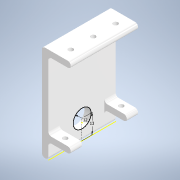
# Autodesk Inventor part: BearingBracket
Saved by Autodesk Inventor 2021 (Build 250183000, 183)
## iProperties
Created: 2021-05-21
Part Number: BearingBracket
Material: PC/ABS Plastic
Document SubType Name: Modeling
Designer: sami8
Density: 0.357273 g/cm^3
Appearance: Smooth - White
Author: sami8
Autodesk Inventor part; units mm, degrees
ref_plane "YZ Plane" through (0, 0, 0) normal (1, 0, 0) x (0, 1, 0)
ref_plane "XZ Plane" through (0, 0, 0) normal (0, 1, 0) x (-1, 0, 0)
ref_plane "XY Plane" through (0, 0, 0) normal (0, 0, 1) x (1, 0, 0)
sketch "Sketch1" plane through (0, 0, 0) normal (0, 0, 1) x (1, 0, 0)
  line L0 (0, 0) -> (15, 0)
  line L1 (15, 0) -> (15, 4)
  line L2 (15, 4) -> (0, 4)
  line L3 (0, 4) -> (0, 0)
  line L4 (0, 53.5) -> (15, 53.5)
  line L5 (15, 53.5) -> (15, 49.5)
  line L6 (15, 49.5) -> (0, 49.5)
  line L7 (0, 49.5) -> (0, 53.5)
  line L8 (0, 53.5) -> (-4.3, 53.5)
  line L9 (-4.3, 53.5) -> (-4.3, -10.5)
  line L10 (-4.3, -10.5) -> (0, -10.5)
  line L11 (0, -10.5) -> (0, 53.5)
  point P0 (0, 49.5)
  dimension "d0" = 15
  dimension "d1" = 4
  dimension "d2" = 15
  dimension "d3" = 4
  dimension "d4" = 45.5
  dimension "d5" = 4.3
  dimension "d6" = 64
  constraints: 24 end point, 6 parallel, 3 horizontal, 3 perpendicular, 1 point on line
  measures "d0" distance of L2.end L1.end
  measures "d1" distance of L1.end L0.end
  measures "d2" distance of L5.end L6.end
  measures "d3" distance of L4.end L5.end
  measures "d4" distance between parallel lines of L6 L2
  measures "d5" distance of L10.end L9.end
  measures "d6" distance between parallel lines of L8 L10
extrude "Extrusion1" add sketch "Sketch1" along normal mid plane 45
extrude "Extrusion2" cut sketch "Sketch1" along normal mid plane 30 contours L3 L2 L1 L0
sketch "Sketch3" plane through (0, 49.5, 22.5) normal (0, -1, 0) x (1, 0, 0)
  line L0 (0, 0) -> (15, 0) projected
  line L1 (7.5, 0) -> (7.5, -45)
  line L2 (15, -45) -> (0, -45) projected
  circle A0 centre (7.5, -3.75) radius 1.55
  circle A1 centre (7.5, -7.5) radius 1.55
  circle A2 centre (7.5, -22.5) radius 1.55
  circle A3 centre (7.5, -37.5) radius 1.55
  circle A4 centre (7.5, -41.25) radius 1.55
  line L3 (0, 0) -> (15, 0) projected
  line L4 (15, -45) -> (0, -45) projected
  line L5 (15, -45) -> (15, 0) projected
  point P0 (0, -22.5)
  dimension "d11" = 3.1
  dimension "d12" = 3.1
  dimension "d13" = 3.1
  dimension "d14" = 3.1
  dimension "d15" = 3.1
  dimension "d16" = 3.75
  dimension "d17" = 7.5
  dimension "d18" = 3.75
  dimension "d19" = 7.5
  dimension "d20" = 7.5
  constraints: 5 centre point, 4 point on line, 3 midpoint, 2 end point
  measures "d11" diameter of A0
  measures "d12" diameter of A1
  measures "d13" diameter of A2
  measures "d14" diameter of A3
  measures "d15" diameter of A4
  measures "d16" distance from line of L0 A0.centre
  measures "d17" distance from line of A1.centre L0
  measures "d18" distance from line of L2 A4.centre
  measures "d19" distance from line of L2 A3.centre
  measures "d20" distance between parallel lines of L5 L1
extrude "Extrusion3" cut sketch "Sketch3" along normal through all contours A0 L1 | L1 A0 | A4 L1 | L1 A4
extrude "Extrusion4" cut sketch "Sketch3" against normal through all contours A1 L1 | L1 A1 | A2 L1 | L1 A2 | A3 L1 | L1 A3
sketch "Sketch4" plane through (0, 4, -22.5) normal (1, 0, 0) x (0, 0, -1)
  circle A0 centre (-22.5, -1.5) radius 6
  line L0 (-45, -14.5) -> (0, -14.5) projected
  line L1 (-22.5, -1.5) -> (-22.5, -14.5) construction
  point P0 (-22.5, -4)
  dimension "d29" = 12
  dimension "d40" = 13
  constraints: 2 end point, 1 centre point, 1 midpoint, 1 vertical
  measures "d29" diameter of A0
  measures "d40" distance of L1.start L1.end
extrude "Extrusion6" cut sketch "Sketch4" against normal through all
fillet "Fillet1" radius 2 14 edges at (0, 49.5, 0) (15, 49.5, 0) (15, 53.5, 0) (-4.3, 53.5, 0) (0, 4, 18.75) (0, 4, -18.75) (15, 4, -18.75) (15, 0, -18.75) (15, 4, 18.75) (15, 0, 18.75) (0, -10.5, 0) (0, 0, 18.75) (0, 0, -18.75) (-4.3, -10.5, 0)
body "Solid1"
